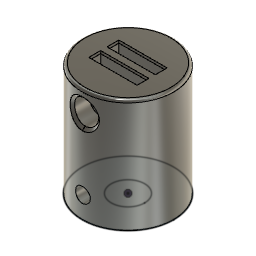
Adaptateur_paralenz_caisson_moteur (Autodesk Fusion 360 design; units mm, degrees)
Autodesk Fusion 360 part; units mm, degrees
sketch "Esquisse1" plane through (0, 0, 0) normal (0, 0, 1) x (1, 0, 0)
  circle A0 centre (0, 0) radius 17
  circle A1 centre (0, 0) radius 6.2
  dimension "d1" = 34
  dimension "d2" = 12.4
  constraint coincident A0.centre A1.centre
  constraint concentric A0 A1
  measures "d1" diameter of A0
  measures "d2" diameter of A1
extrude "Extrusion1" add sketch "Esquisse1" along normal blind 22.2 contours A0 | A1
extrude "Extrusion2" cut sketch "Esquisse1" along normal blind 18.5 contours A1
hole "Perçage1" at (0, -17, 8) direction (0, 1, 0) diameter 5.5 depth 17 tip angle 180
ref_plane "Plan de construction1" through (0, -13, 0) normal (0, 1, 0) x (0, 0, 1)
sketch "Esquisse2" plane through (0, -13, 0) normal (0, 1, 0) x (1, 0, 0)
  line L0 (-4.1, 0) -> (4.1, 0)
  line L1 (4.1, 0) -> (4.1, -8)
  line L2 (-4.1, -8) -> (-4.1, 0)
  line L3 (-4.1, -10.3671) -> (0, -12.7343)
  line L4 (0, -12.7343) -> (4.1, -10.3671)
  line L5 (-4.1, -10.3671) -> (-4.1, -8)
  line L6 (4.1, -10.3671) -> (4.1, -8)
  point P0 (0, -8)
  dimension "d12" = 8.2
  dimension "d13" = 4.1
  dimension "d14" = 8
  constraint horizontal L0
  constraint vertical L1
  constraint vertical L2
  constraint parallel L2 L5
  constraint parallel L2 L6
  measures "d12" distance of L0.start L0.end
  measures "d13" distance of L1 origin
  measures "d14" distance of L0.start L2.start
extrude "Extrusion3" cut sketch "Esquisse2" along normal blind 4.9
extrude "Extrusion4" add 1 faces at (1.6321, -3.8543, 22.2) along direction (0, 0, 1) blind 20
sketch "Esquisse5" plane through (0, 0, 42.2) normal (0, 0, 1) x (-1, 0, 0)
  circle A0 centre (0, 0) radius 17
  line L0 (8.5, 5.1) -> (-8.5, 5.1)
  line L1 (-8.5, 5.1) -> (-8.5, 1.7)
  line L2 (-8.5, 1.7) -> (8.5, 1.7)
  line L3 (8.5, 1.7) -> (8.5, 5.1)
  line L4 (11.5333, 0) -> (-9, 0) construction
  line L5 (-8.5, -1.7) -> (8.5, -1.7)
  line L6 (8.5, -1.7) -> (8.5, -5.1)
  line L7 (8.5, -5.1) -> (-8.5, -5.1)
  line L8 (-8.5, -5.1) -> (-8.5, -1.7)
  dimension "d20" = 17
  dimension "d21" = 3.4
  dimension "d22" = 8.5
  dimension "d23" = 1.7
  constraint horizontal L0
  constraint vertical L1
  constraint horizontal L2
  constraint vertical L3
  constraint parallel L2 L4
  constraint symmetric L0.start L4 L6.end
  constraint symmetric L0.end L4 L7.end
  constraint symmetric L1.end L4 L5.start
  constraint symmetric L2.end L4 L5.end
  measures "d20" distance of L0.start L0.end
  measures "d21" distance of L0.start L2.end
  measures "d22" distance of A0.centre L1
  measures "d23" distance of A0.centre L2
extrude "Extrusion5" cut sketch "Esquisse5" against normal blind 16.5 contours L0 L1 L2 L3 | L5 L6 L7 L8
hole "Perçage2" at (0, -17, 34.2) direction (0, 1, 0) diameter 5.5 depth 41 tip angle 180 counterbore diameter 9 counterbore depth 7
sketch "Esquisse6" plane through (0, 0, 0) normal (0, 1, 0) x (1, 0, 0)
ref_plane "Plan de construction2" through (0, 17, 0) normal (0, 1, 0) x (0, 0, 1)
sketch "Esquisse7" plane through (0, 17, 0) normal (0, 1, 0) x (1, 0, 0)
  line L0 (0.2093, -36.942) -> (6.8092, -36.4383) construction
  circle A0 centre (0, -34.2) radius 2.75
  line L1 (0.2093, -36.942) -> (0, -34.2) construction
  line L2 (-4.1594, -31.7062) -> (-4.2394, -36.5552)
  line L3 (-4.2394, -36.5552) -> (-0.08, -39.0491)
  line L4 (-0.08, -39.0491) -> (4.1594, -36.6938)
  line L5 (4.1594, -36.6938) -> (4.2394, -31.8448)
  line L6 (4.2394, -31.8448) -> (0.08, -29.3509)
  line L7 (0.08, -29.3509) -> (-4.1594, -31.7062)
  point P0 (0, -34.2)
  dimension "d33" = 4.2
  constraint tangent L0 A0
  constraint coincident P0 A0.centre
  constraint perpendicular L0 L1
  measures "d33" distance of P0 L7
extrude "Extrusion6" cut sketch "Esquisse7" against normal blind 5
chamfer "Chanfrein1" distance 0.5 angle 45 8 edges at (0, 1.7, 42.2) (8.5, 3.4, 42.2) (0, 5.1, 42.2) (-8.5, 3.4, 42.2) (0, -1.7, 42.2) (-8.5, -3.4, 42.2) (0, -5.1, 42.2) (8.5, -3.4, 42.2)
chamfer "Chanfrein2" distance 1 angle 45 2 edges at (4.5, -16.3936, 34.2) (-4.5, -16.3936, 34.2)
chamfer "Chanfrein3" distance 1 angle 45 6 edges at (2.1763, 16.8601, 30.6078) (4.1994, 16.4732, 34.2685) (2.056, 16.8752, 37.8624) (-2.1763, 16.8601, 37.7922) (-4.1994, 16.4732, 34.1315) (-2.056, 16.8752, 30.5376)
fillet "Congé1" radius 1 1 edges at (-15.8496, -6.1475, 42.2)
equation "d13 = d12 / 2"
equation "d22 = d20 / 2"
equation "d23 = ( 3.4 / 2 ) * 1 mm"
